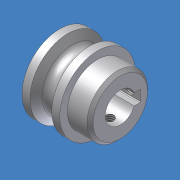
# Autodesk Inventor part: MBR18-2-N8
Saved by Autodesk Inventor 2015 (Build 190159000, 159)
## iProperties
Category: PARTsolutions
Created: 2015-02-25
Part Number: MBR18-2-N8
Catalog Web Link: www.cadenas.de
Description: MBRF, MBRFM, MBRFA, MBR, MBRM, MBRS, MBRA - Pulleys for Round Belts - Set Screw Type - U Groove
Document SubType Name: Modeling
Designer: PARTsolutions
Material: Generic
Density: 1 g/cm^3
Appearance: RGB(175,175,175)
NB: MBR18-2-N8
NN: MBRF, MBRFM, MBRFA, MBR, MBRM, MBRS, MBRA
NT: Pulleys for Round Belts - Set Screw Type - U Groove
NBSYN: $PN.
LINA: MBR18-2-N8
PN: MBR18-2-N8
TYPE: MBR
SHP: 2
SHP1: '1','A Shape','2','B Shape'
MAT: 1
MAT1: '1', 'S45C', '2', 'SUS304', '3', 'A5052'
ST: 1
ST0: '1','Black Oxide','2','Electroless Nickel Plating'
SHS: N
SHS1: 'H','Round Hole','P','Round Hole+Tap','N','New JIS Key Groove Hole+Tap','C','Old JIS Key Groove Hole+Tap'
R: 2.0
PD: 18
PDO: 18,23,28,30,40,45,48,60,80
PDO1: 18,23,28,30,40,45,48,60,80
PDO2: 45,48,60,80
PDO3: 18,23,28,30,40,45,48,60,80
PDO4: 23,28,30,40,45,48,60,80
ID: 8
ID0: '8','8'
ID1: 8.00
D1: 20
D2: 14
T: 10
L: 16
LL: 3
D: 16
MM: M3
MMM: 3
MMMIN: 2.459
ALT: MBR18-2-N8
WW: 3.000
DD: 1.400
CBD: 4
ALT1ALG: '','w/o DC (Outer Diameter Cut)','-DC','with DC (Outer Diameter Cut)'
DC: 0.0
BB: 3
TT: 1.4
Z: 2
TIF: 6
NAV: 0
KT: DUMMY
CreationOption_UseAsmMates: 0
SUPPLIER: Misumi
ARTICLENO: MBR18-2-N8
BOMINFO: MBR18-2-N8
CREATOR: CADENAS GmbH
PSOL_IDENT_0: {\\10.0.0.236\data_v8\23d-libs\misumi\metric\52_belts_pulleys\mbra.prj},222 {VTYP=3D},{NB=MBR18-2-N8
PSOL_IDENT_1: },{LINA=MBR18-2-N8},{NN=MBRF, MBRFM, MBRFA, MBR, MBRM, MBRS, MBRA},{DATE=13.11.2014 02:11:09},{GEOMD
PSOL_IDENT_2: ATE=02.09.2014 00:00:00},{VERSION=},{LINEID=60},{LINESUBID=-1},{WBVAR=SHP,MAT,ST,SHS,PD,ID,ALT1}  {N
PSOL_IDENT_3: B=MBR18-2-N8},{LINA=MBR18-2-N8},{KT=DUMMY},{PN=MBR18-2-N8},{TYPE=MBR},{SHP=2},{SHP1='1','A Shape','2
PSOL_IDENT_4: ','B Shape'},{MAT=1},{MAT1='1', 'S45C', '2', 'SUS304', '3', 'A5052'},{ST=1},{ST0='1','Black Oxide','
PSOL_IDENT_5: 2','Electroless Nickel Plating'},{SHS=N},{SHS1='H','Round Hole','P','Round Hole+Tap','N','New JIS Ke
PSOL_IDENT_6: y Groove Hole+Tap','C','Old JIS Key Groove Hole+Tap'},{R=2.0},{PD=18},{PDO=18,23,28,30,40,45,48,60,8
PSOL_IDENT_7: 0},{PDO1=18,23,28,30,40,45,48,60,80},{PDO2=45,48,60,80},{PDO3=18,23,28,30,40,45,48,60,80},{PDO4=23,2
PSOL_IDENT_8: 8,30,40,45,48,60,80},{ID=8},{ID0= '8','8' },{ID1=8.00},{D1=20},{D2=14},{T=10},{L=16},{LL=3},{D=16},{
PSOL_IDENT_9: MM=M3},{MMM=3},{MMMIN=2.459},{ALT=MBR18-2-N8},{WW=3},{DD=1.4},{CBD=4},{ALT1=},{ALT1ALG='','w/o DC (O
PSOL_IDENT_10: uter Diameter Cut)','-DC','with DC (Outer Diameter Cut)'},{DC=0.0},{BB=3},{TT=1.4},{Z=2},{TIF=6},{NA
PSOL_IDENT_11: V=0}
Title: MBR18-2-N8
Author: Cadenas PARTsolutions
Comments: Pulleys for Round Belts - Set Screw Type - U Groove
Autodesk Inventor part; units mm, degrees
ref_plane "YZ Plane" through (0, 0, 0) normal (1, 0, 0) x (0, 1, 0)
ref_plane "XZ Plane" through (0, 0, 0) normal (0, 1, 0) x (-1, 0, 0)
ref_plane "XY Plane" through (0, 0, 0) normal (0, 0, 1) x (1, 0, 0)
sketch "Sketch_2" plane through (0, 0, 0) normal (0, 0, 1) x (1, 0, 0)
  line L0 (11, 0) -> (-5, 0)
  line L1 (-5, 10) -> (-5, 4)
  line L2 (-5, 4) -> (11, 4)
  line L3 (11, 4) -> (11, 7.2)
  line L4 (11, 7.2) -> (10.2, 8)
  line L5 (10.2, 8) -> (5, 8)
  line L6 (5, 8) -> (5, 10)
  line L7 (5, 10) -> (2.8868, 10)
  line L8 (2.8868, 10) -> (1.7321, 8)
  arc A0 (-1.7321, 8) -> (1.7321, 8) centre (0, 9) ccw
  line L9 (-1.7321, 8) -> (-2.8868, 10)
  line L10 (-2.8868, 10) -> (-5, 10)
  constraints: 22 end point, 2 point on circle, 1 centre point
revolve "Revolution1" add sketch "Sketch_2" angle 360 about axis through (11, 0, 0) along (1, 0, 0)
sketch "Sketch_4" plane through (-5, 0, 0) normal (1, 0, 0) x (0, 0, -1)
  line L0 (-1.5, 2.6) -> (1.5, 2.6)
  line L1 (1.5, 2.6) -> (1.5, 5.2)
  arc A0 (1.5, 5.2) -> (1.3, 5.4) centre (1.3, 5.2) ccw
  line L2 (1.3, 5.4) -> (-1.3, 5.4)
  arc A1 (-1.3, 5.4) -> (-1.5, 5.2) centre (-1.3, 5.2) ccw
  line L3 (-1.5, 5.2) -> (-1.5, 2.6)
  constraints: 8 end point, 4 point on circle, 2 centre point
extrude "Extrusion1" cut sketch "Sketch_4" along normal blind 30
sketch "Sketch_5" plane through (0, 0, 0) normal (0, 0, 1) x (1, 0, 0)
  line L0 (8, 5.4) -> (8, 8)
  line L1 (8, 8) -> (9.5, 8)
  line L2 (9.5, 8) -> (9.2295, 7.7295)
  line L3 (9.2295, 7.7295) -> (9.2295, 5.4)
  line L4 (9.2295, 5.4) -> (8, 5.4)
  line L5 (8, 5.4) -> (8, 8)
  constraints: 12 end point
revolve "Revolution2" cut sketch "Sketch_5" angle 360 about axis through (8, 5.4, 0) along (0, -1, 0)
thread "Thread1" size "M3x0.5" class "6H" standard "ISO Metric profile" full length
sketch "Sketch_8" plane through (0, 0, 0) normal (0, 1, 0) x (-1, 0, 0)
  line L0 (-8, -3) -> (-8, -8)
  line L1 (-8, -8) -> (-9.5, -8)
  line L2 (-9.5, -8) -> (-9.2295, -7.7295)
  line L3 (-9.2295, -7.7295) -> (-9.2295, -3)
  line L4 (-9.2295, -3) -> (-8, -3)
  line L5 (-8, -3) -> (-8, -8)
  constraints: 12 end point
revolve "Revolution3" cut sketch "Sketch_8" angle 360 about axis through (8, 0, -3) along (0, 0, 1)
thread "Thread2" size "M3x0.5" class "6H" standard "ISO Metric profile" full length
body "Solid1"
